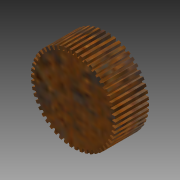
# Autodesk Inventor part: Small Continuous Servo Gear
Saved by Autodesk Inventor 2016 SP2 (Build 200236200, 236)
## iProperties
Created: 2015-07-13
Part Number: Small Continuous Servo Gear
Material: Generic
Document SubType Name: Modeling
Designer: Jared
Density: 1 g/cm^3
Appearance: Rust
Author: Jared
Autodesk Inventor part; units mm, degrees
ref_plane "YZ Plane" through (0, 0, 0) normal (1, 0, 0) x (0, 1, 0)
ref_plane "XZ Plane" through (0, 0, 0) normal (0, 1, 0) x (-1, 0, 0)
ref_plane "XY Plane" through (0, 0, 0) normal (0, 0, 1) x (1, 0, 0)
sketch "Sketch1" plane through (0, 0, 0) normal (0, 1, 0) x (-1, 0, 0)
  circle A0 centre (0, 0) radius 2.5
  dimension "d0" = 5
  constraints: 1 centre point, 1 coincident
  measures "d0" diameter of A0
extrude "Extrusion1" add sketch "Sketch1" along normal blind 2
sketch "Sketch2" plane through (0, 2, 0) normal (0, 1, 0) x (1, 0, 0)
  line L0 (0, 2.3) -> (-0.05, 2.3)
  line L1 (-0.05, 2.3) -> (-0.085, 2.4986)
  line L2 (0, 0) -> (0, 2.3)
  line L3 (0, 2.3) -> (0.05, 2.3)
  line L4 (0.05, 2.3) -> (0.085, 2.4986)
  arc A0 (0.085, 2.4986) -> (-0.085, 2.4986) centre (0, 0) ccw
  line L5 (-0.2883, 2.2819) -> (-0.3379, 2.2756)
  line L6 (-0.3379, 2.2756) -> (-0.3975, 2.4682)
  line L7 (-0.2387, 2.2881) -> (-0.2288, 2.4895)
  line L8 (-0.2883, 2.2819) -> (-0.2387, 2.2881)
  arc A1 (-0.2288, 2.4895) -> (-0.3975, 2.4682) centre (0, 0) ccw
  line L9 (-0.572, 2.2277) -> (-0.6204, 2.2153)
  line L10 (-0.6204, 2.2153) -> (-0.7037, 2.3989)
  line L11 (-0.5236, 2.2402) -> (-0.539, 2.4412)
  line L12 (-0.572, 2.2277) -> (-0.5236, 2.2402)
  arc A2 (-0.539, 2.4412) -> (-0.7037, 2.3989) centre (0, 0) ccw
  line L13 (-0.8467, 2.1385) -> (-0.8932, 2.1201)
  line L14 (-0.8932, 2.1201) -> (-0.9988, 2.2918)
  line L15 (-0.8002, 2.1569) -> (-0.8407, 2.3544)
  line L16 (-0.8467, 2.1385) -> (-0.8002, 2.1569)
  arc A3 (-0.8407, 2.3544) -> (-0.9988, 2.2918) centre (0, 0) ccw
  line L17 (-1.108, 2.0155) -> (-1.1518, 1.9914)
  line L18 (-1.1518, 1.9914) -> (-1.2782, 2.1485)
  line L19 (-1.0642, 2.0396) -> (-1.1292, 2.2305)
  line L20 (-1.108, 2.0155) -> (-1.0642, 2.0396)
  arc A4 (-1.1292, 2.2305) -> (-1.2782, 2.1485) centre (0, 0) ccw
  line L21 (-1.3519, 1.8607) -> (-1.3924, 1.8313)
  line L22 (-1.3924, 1.8313) -> (-1.5374, 1.9714)
  line L23 (-1.3115, 1.8901) -> (-1.3998, 2.0713)
  line L24 (-1.3519, 1.8607) -> (-1.3115, 1.8901)
  arc A5 (-1.3998, 2.0713) -> (-1.5374, 1.9714) centre (0, 0) ccw
  line L25 (-1.5745, 1.6766) -> (-1.6109, 1.6424)
  line L26 (-1.6109, 1.6424) -> (-1.7723, 1.7632)
  line L27 (-1.538, 1.7109) -> (-1.6484, 1.8796)
  line L28 (-1.5745, 1.6766) -> (-1.538, 1.7109)
  arc A6 (-1.6484, 1.8796) -> (-1.7723, 1.7632) centre (0, 0) ccw
  line L29 (-1.7722, 1.4661) -> (-1.8041, 1.4275)
  line L30 (-1.8041, 1.4275) -> (-1.9794, 1.5271)
  line L31 (-1.7403, 1.5046) -> (-1.871, 1.6581)
  line L32 (-1.7722, 1.4661) -> (-1.7403, 1.5046)
  arc A7 (-1.871, 1.6581) -> (-1.9794, 1.5271) centre (0, 0) ccw
  line L33 (-1.942, 1.2324) -> (-1.9687, 1.1902)
  line L34 (-1.9687, 1.1902) -> (-2.1551, 1.267)
  line L35 (-1.9152, 1.2746) -> (-2.064, 1.4106)
  line L36 (-1.942, 1.2324) -> (-1.9152, 1.2746)
  arc A8 (-2.064, 1.4106) -> (-2.1551, 1.267) centre (0, 0) ccw
  line L37 (-2.0811, 0.9793) -> (-2.1024, 0.9341)
  line L38 (-2.1024, 0.9341) -> (-2.297, 0.9869)
  line L39 (-2.0598, 1.0245) -> (-2.2246, 1.1408)
  line L40 (-2.0811, 0.9793) -> (-2.0598, 1.0245)
  arc A9 (-2.2246, 1.1408) -> (-2.297, 0.9869) centre (0, 0) ccw
  line L41 (-2.1874, 0.7107) -> (-2.2029, 0.6632)
  line L42 (-2.2029, 0.6632) -> (-2.4025, 0.6912)
  line L43 (-2.172, 0.7583) -> (-2.35, 0.8529)
  line L44 (-2.1874, 0.7107) -> (-2.172, 0.7583)
  arc A10 (-2.35, 0.8529) -> (-2.4025, 0.6912) centre (0, 0) ccw
  line L45 (-2.2593, 0.431) -> (-2.2686, 0.3819)
  line L46 (-2.2686, 0.3819) -> (-2.4702, 0.3847)
  line L47 (-2.2499, 0.4801) -> (-2.4384, 0.5517)
  line L48 (-2.2593, 0.431) -> (-2.2499, 0.4801)
  arc A11 (-2.4384, 0.5517) -> (-2.4702, 0.3847) centre (0, 0) ccw
  line L49 (-2.2955, 0.1444) -> (-2.2986, 0.0945)
  line L50 (-2.2986, 0.0945) -> (-2.499, 0.072)
  line L51 (-2.2923, 0.1943) -> (-2.4883, 0.2417)
  line L52 (-2.2955, 0.1444) -> (-2.2923, 0.1943)
  arc A12 (-2.4883, 0.2417) -> (-2.499, 0.072) centre (0, 0) ccw
  line L53 (-2.2955, -0.1444) -> (-2.2923, -0.1943)
  line L54 (-2.2923, -0.1943) -> (-2.4883, -0.2417)
  line L55 (-2.2986, -0.0945) -> (-2.499, -0.072)
  line L56 (-2.2955, -0.1444) -> (-2.2986, -0.0945)
  arc A13 (-2.499, -0.072) -> (-2.4883, -0.2417) centre (0, 0) ccw
  line L57 (-2.2593, -0.431) -> (-2.2499, -0.4801)
  line L58 (-2.2499, -0.4801) -> (-2.4384, -0.5517)
  line L59 (-2.2686, -0.3819) -> (-2.4702, -0.3847)
  line L60 (-2.2593, -0.431) -> (-2.2686, -0.3819)
  arc A14 (-2.4702, -0.3847) -> (-2.4384, -0.5517) centre (0, 0) ccw
  line L61 (-2.1874, -0.7107) -> (-2.172, -0.7583)
  line L62 (-2.172, -0.7583) -> (-2.35, -0.8529)
  line L63 (-2.2029, -0.6632) -> (-2.4025, -0.6912)
  line L64 (-2.1874, -0.7107) -> (-2.2029, -0.6632)
  arc A15 (-2.4025, -0.6912) -> (-2.35, -0.8529) centre (0, 0) ccw
  line L65 (-2.0811, -0.9793) -> (-2.0598, -1.0245)
  line L66 (-2.0598, -1.0245) -> (-2.2246, -1.1408)
  line L67 (-2.1024, -0.9341) -> (-2.297, -0.9869)
  line L68 (-2.0811, -0.9793) -> (-2.1024, -0.9341)
  arc A16 (-2.297, -0.9869) -> (-2.2246, -1.1408) centre (0, 0) ccw
  line L69 (-1.942, -1.2324) -> (-1.9152, -1.2746)
  line L70 (-1.9152, -1.2746) -> (-2.064, -1.4106)
  line L71 (-1.9687, -1.1902) -> (-2.1551, -1.267)
  line L72 (-1.942, -1.2324) -> (-1.9687, -1.1902)
  arc A17 (-2.1551, -1.267) -> (-2.064, -1.4106) centre (0, 0) ccw
  line L73 (-1.7722, -1.4661) -> (-1.7403, -1.5046)
  line L74 (-1.7403, -1.5046) -> (-1.871, -1.6581)
  line L75 (-1.8041, -1.4275) -> (-1.9794, -1.5271)
  line L76 (-1.7722, -1.4661) -> (-1.8041, -1.4275)
  arc A18 (-1.9794, -1.5271) -> (-1.871, -1.6581) centre (0, 0) ccw
  line L77 (-1.5745, -1.6766) -> (-1.538, -1.7109)
  line L78 (-1.538, -1.7109) -> (-1.6484, -1.8796)
  line L79 (-1.6109, -1.6424) -> (-1.7723, -1.7632)
  line L80 (-1.5745, -1.6766) -> (-1.6109, -1.6424)
  arc A19 (-1.7723, -1.7632) -> (-1.6484, -1.8796) centre (0, 0) ccw
  line L81 (-1.3519, -1.8607) -> (-1.3115, -1.8901)
  line L82 (-1.3115, -1.8901) -> (-1.3998, -2.0713)
  line L83 (-1.3924, -1.8313) -> (-1.5374, -1.9714)
  line L84 (-1.3519, -1.8607) -> (-1.3924, -1.8313)
  arc A20 (-1.5374, -1.9714) -> (-1.3998, -2.0713) centre (0, 0) ccw
  line L85 (-1.108, -2.0155) -> (-1.0642, -2.0396)
  line L86 (-1.0642, -2.0396) -> (-1.1292, -2.2305)
  line L87 (-1.1518, -1.9914) -> (-1.2782, -2.1485)
  line L88 (-1.108, -2.0155) -> (-1.1518, -1.9914)
  arc A21 (-1.2782, -2.1485) -> (-1.1292, -2.2305) centre (0, 0) ccw
  line L89 (-0.8467, -2.1385) -> (-0.8002, -2.1569)
  line L90 (-0.8002, -2.1569) -> (-0.8407, -2.3544)
  line L91 (-0.8932, -2.1201) -> (-0.9988, -2.2918)
  line L92 (-0.8467, -2.1385) -> (-0.8932, -2.1201)
  arc A22 (-0.9988, -2.2918) -> (-0.8407, -2.3544) centre (0, 0) ccw
  line L93 (-0.572, -2.2277) -> (-0.5236, -2.2402)
  line L94 (-0.5236, -2.2402) -> (-0.539, -2.4412)
  line L95 (-0.6204, -2.2153) -> (-0.7037, -2.3989)
  line L96 (-0.572, -2.2277) -> (-0.6204, -2.2153)
  arc A23 (-0.7037, -2.3989) -> (-0.539, -2.4412) centre (0, 0) ccw
  line L97 (-0.2883, -2.2819) -> (-0.2387, -2.2881)
  line L98 (-0.2387, -2.2881) -> (-0.2288, -2.4895)
  line L99 (-0.3379, -2.2756) -> (-0.3975, -2.4682)
  line L100 (-0.2883, -2.2819) -> (-0.3379, -2.2756)
  arc A24 (-0.3975, -2.4682) -> (-0.2288, -2.4895) centre (0, 0) ccw
  line L101 (0, -2.3) -> (0.05, -2.3)
  line L102 (0.05, -2.3) -> (0.085, -2.4986)
  line L103 (-0.05, -2.3) -> (-0.085, -2.4986)
  line L104 (0, -2.3) -> (-0.05, -2.3)
  arc A25 (-0.085, -2.4986) -> (0.085, -2.4986) centre (0, 0) ccw
  line L105 (0.2883, -2.2819) -> (0.3379, -2.2756)
  line L106 (0.3379, -2.2756) -> (0.3975, -2.4682)
  line L107 (0.2387, -2.2881) -> (0.2288, -2.4895)
  line L108 (0.2883, -2.2819) -> (0.2387, -2.2881)
  arc A26 (0.2288, -2.4895) -> (0.3975, -2.4682) centre (0, 0) ccw
  line L109 (0.572, -2.2277) -> (0.6204, -2.2153)
  line L110 (0.6204, -2.2153) -> (0.7037, -2.3989)
  line L111 (0.5236, -2.2402) -> (0.539, -2.4412)
  line L112 (0.572, -2.2277) -> (0.5236, -2.2402)
  arc A27 (0.539, -2.4412) -> (0.7037, -2.3989) centre (0, 0) ccw
  line L113 (0.8467, -2.1385) -> (0.8932, -2.1201)
  line L114 (0.8932, -2.1201) -> (0.9988, -2.2918)
  line L115 (0.8002, -2.1569) -> (0.8407, -2.3544)
  line L116 (0.8467, -2.1385) -> (0.8002, -2.1569)
  arc A28 (0.8407, -2.3544) -> (0.9988, -2.2918) centre (0, 0) ccw
  line L117 (1.108, -2.0155) -> (1.1518, -1.9914)
  line L118 (1.1518, -1.9914) -> (1.2782, -2.1485)
  line L119 (1.0642, -2.0396) -> (1.1292, -2.2305)
  line L120 (1.108, -2.0155) -> (1.0642, -2.0396)
  arc A29 (1.1292, -2.2305) -> (1.2782, -2.1485) centre (0, 0) ccw
  line L121 (1.3519, -1.8607) -> (1.3924, -1.8313)
  line L122 (1.3924, -1.8313) -> (1.5374, -1.9714)
  line L123 (1.3115, -1.8901) -> (1.3998, -2.0713)
  line L124 (1.3519, -1.8607) -> (1.3115, -1.8901)
  arc A30 (1.3998, -2.0713) -> (1.5374, -1.9714) centre (0, 0) ccw
  line L125 (1.5745, -1.6766) -> (1.6109, -1.6424)
  line L126 (1.6109, -1.6424) -> (1.7723, -1.7632)
  line L127 (1.538, -1.7109) -> (1.6484, -1.8796)
  line L128 (1.5745, -1.6766) -> (1.538, -1.7109)
  arc A31 (1.6484, -1.8796) -> (1.7723, -1.7632) centre (0, 0) ccw
  line L129 (1.7722, -1.4661) -> (1.8041, -1.4275)
  line L130 (1.8041, -1.4275) -> (1.9794, -1.5271)
  line L131 (1.7403, -1.5046) -> (1.871, -1.6581)
  line L132 (1.7722, -1.4661) -> (1.7403, -1.5046)
  arc A32 (1.871, -1.6581) -> (1.9794, -1.5271) centre (0, 0) ccw
  line L133 (1.942, -1.2324) -> (1.9687, -1.1902)
  line L134 (1.9687, -1.1902) -> (2.1551, -1.267)
  line L135 (1.9152, -1.2746) -> (2.064, -1.4106)
  line L136 (1.942, -1.2324) -> (1.9152, -1.2746)
  arc A33 (2.064, -1.4106) -> (2.1551, -1.267) centre (0, 0) ccw
  line L137 (2.0811, -0.9793) -> (2.1024, -0.9341)
  line L138 (2.1024, -0.9341) -> (2.297, -0.9869)
  line L139 (2.0598, -1.0245) -> (2.2246, -1.1408)
  line L140 (2.0811, -0.9793) -> (2.0598, -1.0245)
  arc A34 (2.2246, -1.1408) -> (2.297, -0.9869) centre (0, 0) ccw
  line L141 (2.1874, -0.7107) -> (2.2029, -0.6632)
  line L142 (2.2029, -0.6632) -> (2.4025, -0.6912)
  line L143 (2.172, -0.7583) -> (2.35, -0.8529)
  line L144 (2.1874, -0.7107) -> (2.172, -0.7583)
  arc A35 (2.35, -0.8529) -> (2.4025, -0.6912) centre (0, 0) ccw
  line L145 (2.2593, -0.431) -> (2.2686, -0.3819)
  line L146 (2.2686, -0.3819) -> (2.4702, -0.3847)
  line L147 (2.2499, -0.4801) -> (2.4384, -0.5517)
  line L148 (2.2593, -0.431) -> (2.2499, -0.4801)
  arc A36 (2.4384, -0.5517) -> (2.4702, -0.3847) centre (0, 0) ccw
  line L149 (2.2955, -0.1444) -> (2.2986, -0.0945)
  line L150 (2.2986, -0.0945) -> (2.499, -0.072)
  line L151 (2.2923, -0.1943) -> (2.4883, -0.2417)
  line L152 (2.2955, -0.1444) -> (2.2923, -0.1943)
  arc A37 (2.4883, -0.2417) -> (2.499, -0.072) centre (0, 0) ccw
  line L153 (2.2955, 0.1444) -> (2.2923, 0.1943)
  line L154 (2.2923, 0.1943) -> (2.4883, 0.2417)
  line L155 (2.2986, 0.0945) -> (2.499, 0.072)
  line L156 (2.2955, 0.1444) -> (2.2986, 0.0945)
  arc A38 (2.499, 0.072) -> (2.4883, 0.2417) centre (0, 0) ccw
  line L157 (2.2593, 0.431) -> (2.2499, 0.4801)
  line L158 (2.2499, 0.4801) -> (2.4384, 0.5517)
  line L159 (2.2686, 0.3819) -> (2.4702, 0.3847)
  line L160 (2.2593, 0.431) -> (2.2686, 0.3819)
  arc A39 (2.4702, 0.3847) -> (2.4384, 0.5517) centre (0, 0) ccw
  line L161 (2.1874, 0.7107) -> (2.172, 0.7583)
  line L162 (2.172, 0.7583) -> (2.35, 0.8529)
  line L163 (2.2029, 0.6632) -> (2.4025, 0.6912)
  line L164 (2.1874, 0.7107) -> (2.2029, 0.6632)
  arc A40 (2.4025, 0.6912) -> (2.35, 0.8529) centre (0, 0) ccw
  line L165 (2.0811, 0.9793) -> (2.0598, 1.0245)
  line L166 (2.0598, 1.0245) -> (2.2246, 1.1408)
  line L167 (2.1024, 0.9341) -> (2.297, 0.9869)
  line L168 (2.0811, 0.9793) -> (2.1024, 0.9341)
  arc A41 (2.297, 0.9869) -> (2.2246, 1.1408) centre (0, 0) ccw
  line L169 (1.942, 1.2324) -> (1.9152, 1.2746)
  line L170 (1.9152, 1.2746) -> (2.064, 1.4106)
  line L171 (1.9687, 1.1902) -> (2.1551, 1.267)
  line L172 (1.942, 1.2324) -> (1.9687, 1.1902)
  arc A42 (2.1551, 1.267) -> (2.064, 1.4106) centre (0, 0) ccw
  line L173 (1.7722, 1.4661) -> (1.7403, 1.5046)
  line L174 (1.7403, 1.5046) -> (1.871, 1.6581)
  line L175 (1.8041, 1.4275) -> (1.9794, 1.5271)
  line L176 (1.7722, 1.4661) -> (1.8041, 1.4275)
  arc A43 (1.9794, 1.5271) -> (1.871, 1.6581) centre (0, 0) ccw
  line L177 (1.5745, 1.6766) -> (1.538, 1.7109)
  line L178 (1.538, 1.7109) -> (1.6484, 1.8796)
  line L179 (1.6109, 1.6424) -> (1.7723, 1.7632)
  line L180 (1.5745, 1.6766) -> (1.6109, 1.6424)
  arc A44 (1.7723, 1.7632) -> (1.6484, 1.8796) centre (0, 0) ccw
  line L181 (1.3519, 1.8607) -> (1.3115, 1.8901)
  line L182 (1.3115, 1.8901) -> (1.3998, 2.0713)
  line L183 (1.3924, 1.8313) -> (1.5374, 1.9714)
  line L184 (1.3519, 1.8607) -> (1.3924, 1.8313)
  arc A45 (1.5374, 1.9714) -> (1.3998, 2.0713) centre (0, 0) ccw
  line L185 (1.108, 2.0155) -> (1.0642, 2.0396)
  line L186 (1.0642, 2.0396) -> (1.1292, 2.2305)
  line L187 (1.1518, 1.9914) -> (1.2782, 2.1485)
  line L188 (1.108, 2.0155) -> (1.1518, 1.9914)
  arc A46 (1.2782, 2.1485) -> (1.1292, 2.2305) centre (0, 0) ccw
  line L189 (0.8467, 2.1385) -> (0.8002, 2.1569)
  line L190 (0.8002, 2.1569) -> (0.8407, 2.3544)
  line L191 (0.8932, 2.1201) -> (0.9988, 2.2918)
  line L192 (0.8467, 2.1385) -> (0.8932, 2.1201)
  arc A47 (0.9988, 2.2918) -> (0.8407, 2.3544) centre (0, 0) ccw
  line L193 (0.572, 2.2277) -> (0.5236, 2.2402)
  line L194 (0.5236, 2.2402) -> (0.539, 2.4412)
  line L195 (0.6204, 2.2153) -> (0.7037, 2.3989)
  line L196 (0.572, 2.2277) -> (0.6204, 2.2153)
  arc A48 (0.7037, 2.3989) -> (0.539, 2.4412) centre (0, 0) ccw
  line L197 (0.2883, 2.2819) -> (0.2387, 2.2881)
  line L198 (0.2387, 2.2881) -> (0.2288, 2.4895)
  line L199 (0.3379, 2.2756) -> (0.3975, 2.4682)
  line L200 (0.2883, 2.2819) -> (0.3379, 2.2756)
  arc A49 (0.3975, 2.4682) -> (0.2288, 2.4895) centre (0, 0) ccw
  dimension "d4" = 0.05
  dimension "d9" = 2.3
  dimension "d10" = 10
  dimension "d16" = 0.1986
  dimension "d25" = 2.5
  dimension "d28" = 360
  constraints: 402 end point, 100 point on circle, 50 centre point, 2 coincident, 2 symmetric about line, 1 vertical, 549 other
  measures "d4" distance of L0.start L0.end
  measures "d9" distance of L2.start L0.start
  measures "d10" angle of L2 L1
  measures "d16" vertical distance of L0.end L1.end
  measures "d25" radius of A0
extrude "Extrusion2" cut sketch "Sketch2" against normal up to next
body "Solid1"
